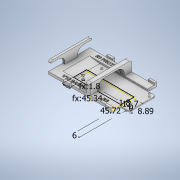
# Autodesk Inventor part: R1 Proto V10 Base
Saved by Autodesk Inventor 2021 (Build 250183000, 183)
## iProperties
Created: 2020-06-07
Part Number: R1 Proto V10 Base
Material: Generic
Document SubType Name: Modeling
Designer: andre
Density: 1 g/cm^3
Appearance: Default
Author: andre
## iProperties of the stored document _3DPrint.ipt
Created: 2020-06-07
Part Number: _3DPrint
Material: Generic
Document SubType Name: Modeling
Designer: andre
Density: 1 g/cm^3
Appearance: Default
Author: andre
Autodesk Inventor part; units mm, degrees
ref_plane "YZ Plane" through (0, 0, 0) normal (1, 0, 0) x (0, 1, 0)
ref_plane "XZ Plane" through (0, 0, 0) normal (0, 1, 0) x (-1, 0, 0)
ref_plane "XY Plane" through (0, 0, 0) normal (0, 0, 1) x (1, 0, 0)
sketch "Sketch1" plane through (0, 0, 0) normal (0, 1, 0) x (-1, 0, 0)
  line L0 (0, 0) -> (62, 0)
  line L1 (62, 0) -> (62, -19.7)
  line L2 (62, -19.7) -> (0, -19.7)
  line L3 (0, -19.7) -> (0, 0)
  dimension "d5" = 62
  dimension "d6" = 19.7
  constraints: 8 end point, 2 parallel, 1 horizontal, 1 perpendicular
  measures "d5" distance of L1.end L2.end
  measures "d6" distance of L0.end L1.end
extrude "Extrusion1" add sketch "Sketch1" along normal blind 2.4
sketch "Sketch3" plane through (-62, 0, 0) normal (0, 0, 1) x (1, 0, 0)
  line L0 (62, 2.4) -> (0, 2.4) projected
  line L1 (62, 0) -> (0, 0) projected
  line L2 (62, 2.4) -> (56, 2.4)
  line L3 (56, 2.4) -> (56, 0)
  line L4 (56, 0) -> (62, 0)
  line L5 (62, 0) -> (62, 2.4)
  line L6 (22, 2.4) -> (22, 0) construction
  line L7 (22, 2.4) -> (16, 2.4)
  line L8 (16, 2.4) -> (16, 0)
  line L9 (16, 0) -> (22, 0)
  line L10 (22, 0) -> (22, 2.4)
  point P0 (62, 0)
  point P1 (22, 0)
  dimension "d9" = 6
  dimension "d13" = 6
  dimension "d14" = 34
  dimension "d79" = 2.4
  constraints: 18 end point, 4 parallel, 4 point on line, 3 perpendicular, 2 horizontal
  measures "d9" distance of L4.end L3.end
  measures "d13" distance of L9.end L8.end
  measures "d14" distance between parallel lines of L3 L6
  measures "d79" distance between parallel lines of L1 L0
extrude "Extrusion2" add sketch "Sketch3" along normal blind 2 contours L5 L1 L3 L0 | L10 L1 L8 L0
ref_plane "Work Plane1" through (0, 0, -19.7) normal (0, 0, -1) x (-1, 0, 0)
sketch "Sketch4" plane through (0, 2.4, 0) normal (0, 1, 0) x (1, 0, 0)
  line L0 (-6, -2) -> (0, -2) projected
  line L1 (-6, -2) -> (0, -2)
  line L2 (0, -2) -> (0, 0)
  line L3 (0, 0) -> (-6, 0)
  line L4 (-6, 0) -> (-6, -2)
  line L5 (-46, -2) -> (-40, -2) projected
  line L6 (-40, 0) -> (-40, -2) projected
  line L7 (-46, -2) -> (-40, -2)
  line L8 (-40, -2) -> (-40, 0)
  line L9 (-40, 0) -> (-46, 0)
  line L10 (-46, 0) -> (-46, -2)
  constraints: 16 end point, 4 parallel, 2 horizontal, 2 perpendicular
extrude "Extrusion3" add sketch "Sketch4" along normal blind 1.6
sketch "Sketch5" plane through (0, 2.4, 0) normal (0, 1, 0) x (1, 0, 0)
  point P0 (0, 0)
sketch "Sketch6" plane through (0, 2.4, 0) normal (0, 1, 0) x (1, 0, 0)
  line L0 (0, 19.7) -> (-62, 19.7) projected
  line L1 (-40, 0) -> (-6, 0) projected
  line L2 (-22, 19.7) -> (-26, 19.7)
  line L3 (-26, 19.7) -> (-26, 0)
  line L4 (-26, 0) -> (-22, 0)
  line L5 (-22, 0) -> (-22, 19.7)
  line L6 (0, 19.7) -> (0, 0) projected
  point P0 (-22, 0)
  point P1 (-26, 19.7)
  dimension "d18" = 4
  dimension "d19" = 22
  constraints: 8 end point, 2 parallel, 2 point on line, 1 horizontal, 1 perpendicular
  measures "d18" distance of L4.end L3.end
  measures "d19" distance between parallel lines of L6 L5
extrude "Extrusion4" add sketch "Sketch6" along normal blind 9.6
sketch "Sketch7" plane through (-22, 2.4, 0) normal (1, 0, 0) x (0, 0, -1)
  point P0 (0, -2.4)
sketch "Sketch8" plane through (-22, 2.4, 0) normal (1, 0, 0) x (0, 0, -1)
  line L0 (19.7, 0) -> (19.7, 9.6) projected
  line L1 (19.7, 0) -> (7, 0)
  line L2 (7, 0) -> (7, 8.1)
  line L3 (7, 8.1) -> (19.7, 8.1)
  line L4 (19.7, 8.1) -> (19.7, 0)
  line L5 (0, 0) -> (0, 9.6) projected
  line L6 (19.7, 0) -> (0, 0) projected
  line L7 (0, 9.6) -> (19.7, 9.6) projected
  point P0 (0, -2.4)
  point P1 (19.7, 8.1)
  dimension "d22" = 19.7
  dimension "d23" = 9.6
  dimension "d24" = 12.7
  dimension "d25" = 8.1
  constraints: 8 end point, 2 parallel, 1 horizontal, 1 perpendicular
  measures "d22" distance between parallel lines of L0 L5
  measures "d23" distance between parallel lines of L6 L7
  measures "d24" distance between parallel lines of L0 L2
  measures "d25" distance between parallel lines of L1 L3
extrude "Extrusion5" cut sketch "Sketch8" against normal blind 37.6 contours L1 L2 L3 L0
ref_plane "Work Plane2" through (-43, 0, -19.7) normal (-1, 0, 0) x (0, 0, 1)
sketch "Sketch12" plane through (0, 2.4, 0) normal (0, 1, 0) x (1, 0, 0)
  line L0 (0, 19.7) -> (0, -2) projected
  line L1 (0, 19.7) -> (-45.34, 19.7)
  line L2 (-45.34, 19.7) -> (-45.34, 7)
  line L3 (-45.34, 7) -> (0, 7)
  line L4 (0, 7) -> (0, 19.7)
  point P0 (0, 0)
  point P1 (0, 7)
  dimension "d41" = 45.34
  dimension "d42" = 12.7
  constraints: 8 end point, 2 parallel, 1 horizontal, 1 perpendicular
  measures "d41" distance between parallel lines of L2 L0
  measures "d42" distance between parallel lines of L1 L3
extrude "Extrusion8" cut sketch "Sketch12" against normal blind 1.4
fillet "Fillet3" radius 2 1 edges at (-24, 12, 0) curvature continuous yes
fillet "Fillet4" radius 7 1 edges at (-24, 10.5, -7) curvature continuous yes
sketch "Sketch13" plane through (0, 1, 0) normal (0, 1, 0) x (1, 0, 0)
  circle A0 centre (6, 10.81) radius 0.9
  circle A1 centre (-39.72, 10.81) radius 0.9
  line L0 (-45.34, 19.7) -> (0, 19.7) projected
  line L1 (0, 19.7) -> (0, 7) projected
  point P0 (0, 0)
  dimension "d48" = 1.8
  dimension "d49" = 1.8
  dimension "d50" = 45.72
  dimension "d51" = 8.89
  dimension "d76" = 6
  dimension "d100" = 0
  constraints: 2 centre point
  measures "d48" diameter of A0
  measures "d49" diameter of A1
  measures "d50" distance of A1.centre A0.centre
  measures "d51" distance from line of L0 A0.centre
  measures "d76" distance from line of L1 A0.centre
  measures "d100" vertical distance of A0.centre A1.centre
extrude "Extrusion9" add sketch "Sketch13" along normal blind 3 contours A0
mirror "Mirror3" about plane through (0, 0, -19.7) normal (0, 0, -1) of "Extrusion4", "Extrusion5", "Fillet4", "Fillet3", "Extrusion1", "Extrusion3", "Extrusion2", "Extrusion9", "Extrusion8"
chamfer "Chamfer1" distance 10 distance2 1.4 1 edges at (-45.34, 2.4, -19.7) measured on face at (-45.84, 2.4, -19.7)
sketch "Sketch15" plane through (0, 2.4, 0) normal (0, 1, 0) x (1, 0, 0)
  line L0 (-57, 38.4) -> (-28, 38.4) construction
  line L1 (-28, 38.4) -> (-28, 33.2) construction
  line L2 (-28, 33.2) -> (-57, 33.2) construction
  line L3 (-57, 33.2) -> (-57, 38.4) construction
  line L4 (-59, 37.4) -> (-59, 2) projected
  line L5 (-26, 2) -> (-26, 37.4) projected
  line L6 (-22, 39.4) -> (-46, 39.4) projected
  line L7 (-55.34, 32.2) -> (0, 32.2) projected
  line L8 (-57, 6) -> (-28, 6) construction
  line L9 (-28, 6) -> (-28, 1) construction
  line L10 (-28, 1) -> (-57, 1) construction
  line L11 (-57, 1) -> (-57, 6) construction
  line L12 (0, 7) -> (-55.34, 7) projected
  line L13 (-40, 0) -> (-46, 0) projected
  line L14 (-15.9129, 6) -> (-6.0871, 6) construction
  line L15 (-6.0871, 6) -> (-6.0871, 1) construction
  line L16 (-6.0871, 1) -> (-15.9129, 1) construction
  line L17 (-15.9129, 1) -> (-15.9129, 6) construction
  line L18 (-22, 2) -> (-22, 37.4) projected
  line L19 (0, 7) -> (0, 0) projected
  spline S0 degree 2 poles (-50.5157, 2) (-50.3394, 2) (-50.1147, 2.1691) (-50.0495, 2.3527) knots 0 0 0 1 2 2 2
  line L20 (-50.0495, 2.3527) -> (-49.2307, 4.5556)
  spline S1 degree 2 poles (-49.2307, 4.5556) (-49.2017, 4.6377) (-49.2017, 4.7174) knots 0 0 0 1 1 1
  spline S2 degree 2 poles (-49.2017, 4.7174) (-49.2041, 4.8454) (-49.3732, 4.9976) (-49.5157, 5) knots 0 0 0 1 2 2 2
  spline S3 degree 2 poles (-49.5157, 5) (-49.6341, 5) (-49.779, 4.8865) (-49.8176, 4.7657) knots 0 0 0 1 2 2 2
  line L21 (-49.8176, 4.7657) -> (-50.4988, 2.6691)
  line L22 (-50.4988, 2.6691) -> (-50.5133, 2.6691)
  line L23 (-50.5133, 2.6691) -> (-51.1969, 4.7585)
  spline S4 degree 2 poles (-51.1969, 4.7585) (-51.2331, 4.8841) (-51.3853, 5) (-51.5085, 5) knots 0 0 0 1 2 2 2
  spline S5 degree 2 poles (-51.5085, 5) (-51.6558, 4.9976) (-51.8273, 4.8406) (-51.8297, 4.7101) knots 0 0 0 1 2 2 2
  spline S6 degree 2 poles (-51.8297, 4.7101) (-51.8297, 4.6232) (-51.8007, 4.5386) knots 0 0 0 1 1 1
  line L24 (-51.8007, 4.5386) -> (-50.9867, 2.3551)
  spline S7 degree 2 poles (-50.9867, 2.3551) (-50.9215, 2.1691) (-50.6944, 2) (-50.5157, 2) knots 0 0 0 1 2 2 2
  spline S8 degree 2 poles (-47.8708, 1.9952) (-47.7331, 1.9976) (-47.5713, 2.1618) (-47.5688, 2.3019) knots 0 0 0 1 2 2 2
  line L25 (-47.5688, 2.3019) -> (-47.5688, 4.6618)
  spline S9 degree 2 poles (-47.5688, 4.6618) (-47.5713, 4.8213) (-47.7524, 5.0024) (-47.9167, 5.0048) knots 0 0 0 1 2 2 2
  spline S10 degree 2 poles (-47.9167, 5.0048) (-48.0085, 5.0048) (-48.1751, 4.9589) (-48.279, 4.8889) knots 0 0 0 1 2 2 2
  line L26 (-48.279, 4.8889) -> (-48.8587, 4.4879)
  spline S11 degree 2 poles (-48.8587, 4.4879) (-48.9287, 4.4372) (-48.9915, 4.3285) (-48.9915, 4.2585) knots 0 0 0 1 2 2 2
  spline S12 degree 2 poles (-48.9915, 4.2585) (-48.9891, 4.1594) (-48.8708, 4.0411) (-48.7766, 4.0411) knots 0 0 0 1 2 2 2
  spline S13 degree 2 poles (-48.7766, 4.0411) (-48.7307, 4.0411) (-48.6558, 4.0652) (-48.6147, 4.0942) knots 0 0 0 1 2 2 2
  line L27 (-48.6147, 4.0942) -> (-48.1872, 4.3937)
  line L28 (-48.1872, 4.3937) -> (-48.1751, 4.3937)
  line L29 (-48.1751, 4.3937) -> (-48.1751, 2.3019)
  spline S14 degree 2 poles (-48.1751, 2.3019) (-48.1727, 2.1618) (-48.0085, 1.9976) (-47.8708, 1.9952) knots 0 0 0 1 2 2 2
  spline S15 degree 2 poles (-45.7597, 1.9734) (-45.3877, 1.9758) (-44.8563, 2.3478) (-44.5713, 3.0314) (-44.5688, 3.5072) knots 0 0 0 1 2 3 3 3
  spline S16 degree 2 poles (-44.5688, 3.5072) (-44.5713, 3.9807) (-44.8563, 4.6594) (-45.3901, 5.0242) (-45.7597, 5.0266) knots 0 0 0 1 2 3 3 3
  spline S17 degree 2 poles (-45.7597, 5.0266) (-46.1292, 5.0242) (-46.663, 4.657) (-46.9505, 3.9783) (-46.9505, 3.5048) knots 0 0 0 1 2 3 3 3
  spline S18 degree 2 poles (-46.9505, 3.5048) (-46.9505, 3.029) (-46.663, 2.3454) (-46.1316, 1.9758) (-45.7597, 1.9734) knots 0 0 0 1 2 3 3 3
  spline S19 degree 2 poles (-45.7597, 2.4638) (-46.0326, 2.4662) (-46.3273, 3) (-46.3297, 3.5048) knots 0 0 0 1 2 2 2
  spline S20 degree 2 poles (-46.3297, 3.5048) (-46.3273, 4.0048) (-46.0278, 4.5338) (-45.7597, 4.5362) knots 0 0 0 1 2 2 2
  spline S21 degree 2 poles (-45.7597, 4.5362) (-45.4891, 4.5338) (-45.192, 4.0048) (-45.1896, 3.5048) knots 0 0 0 1 2 2 2
  spline S22 degree 2 poles (-45.1896, 3.5048) (-45.192, 3) (-45.4867, 2.4662) (-45.7597, 2.4638) knots 0 0 0 1 2 2 2
  line L30 (-43.035, 2.0386) -> (-42.0471, 2.0386)
  spline S23 degree 2 poles (-42.0471, 2.0386) (-41.5737, 2.0435) (-41.0423, 2.4855) (-41.0374, 2.8744) knots 0 0 0 1 2 2 2
  spline S24 degree 2 poles (-41.0374, 2.8744) (-41.0423, 3.1691) (-41.4215, 3.5531) (-41.7258, 3.5821) knots 0 0 0 1 2 2 2
  line L31 (-41.7258, 3.5821) -> (-41.7258, 3.5966)
  spline S25 degree 2 poles (-41.7258, 3.5966) (-41.4867, 3.6377) (-41.1824, 3.9855) (-41.1775, 4.2319) knots 0 0 0 1 2 2 2
  spline S26 degree 2 poles (-41.1775, 4.2319) (-41.18, 4.57) (-41.6534, 4.9565) (-42.0688, 4.9589) knots 0 0 0 1 2 2 2
  line L32 (-42.0688, 4.9589) -> (-43.035, 4.9589)
  spline S27 degree 2 poles (-43.035, 4.9589) (-43.18, 4.9589) (-43.3394, 4.7923) (-43.3394, 4.6425) knots 0 0 0 1 2 2 2
  line L33 (-43.3394, 4.6425) -> (-43.3394, 2.3575)
  spline S28 degree 2 poles (-43.3394, 2.3575) (-43.3394, 2.2053) (-43.18, 2.0386) (-43.035, 2.0386) knots 0 0 0 1 2 2 2
  line L34 (-42.7283, 2.4952) -> (-42.7283, 3.343)
  line L35 (-42.7283, 3.343) -> (-42.2162, 3.343)
  spline S29 degree 2 poles (-42.2162, 3.343) (-41.9457, 3.3406) (-41.6606, 3.128) (-41.6606, 2.9227) knots 0 0 0 1 2 2 2
  spline S30 degree 2 poles (-41.6606, 2.9227) (-41.6606, 2.7126) (-41.9384, 2.4952) (-42.2041, 2.4952) knots 0 0 0 1 2 2 2
  line L36 (-42.2041, 2.4952) -> (-42.7283, 2.4952)
  line L37 (-42.7283, 3.744) -> (-42.7283, 4.5048)
  line L38 (-42.7283, 4.5048) -> (-42.2283, 4.5048)
  spline S31 degree 2 poles (-42.2283, 4.5048) (-42.0109, 4.5024) (-41.779, 4.3116) (-41.779, 4.1353) knots 0 0 0 1 2 2 2
  spline S32 degree 2 poles (-41.779, 4.1353) (-41.779, 3.9493) (-42.0447, 3.7464) (-42.2911, 3.744) knots 0 0 0 1 2 2 2
  line L39 (-42.2911, 3.744) -> (-42.7283, 3.744)
  spline S33 degree 2 poles (-40.494, 2) (-40.3732, 2) (-40.2258, 2.1304) (-40.1848, 2.2754) knots 0 0 0 1 2 2 2
  line L40 (-40.1848, 2.2754) -> (-40.0302, 2.7319)
  line L41 (-40.0302, 2.7319) -> (-38.9771, 2.7319)
  line L42 (-38.9771, 2.7319) -> (-38.8225, 2.2705)
  spline S34 degree 2 poles (-38.8225, 2.2705) (-38.7814, 2.128) (-38.6316, 2) (-38.5036, 2) knots 0 0 0 1 2 2 2
  spline S35 degree 2 poles (-38.5036, 2) (-38.3684, 2.0024) (-38.2017, 2.1594) (-38.1993, 2.2874) knots 0 0 0 1 2 2 2
  spline S36 degree 2 poles (-38.1993, 2.2874) (-38.1993, 2.3333) (-38.2162, 2.4227) (-38.2379, 2.4831) knots 0 0 0 1 2 2 2
  line L43 (-38.2379, 2.4831) -> (-39.0399, 4.6546)
  spline S37 degree 2 poles (-39.0399, 4.6546) (-39.1027, 4.8333) (-39.3273, 5) (-39.506, 5) knots 0 0 0 1 2 2 2
  spline S38 degree 2 poles (-39.506, 5) (-39.6775, 5) (-39.9022, 4.8309) (-39.965, 4.6546) knots 0 0 0 1 2 2 2
  line L44 (-39.965, 4.6546) -> (-40.7621, 2.4831)
  spline S39 degree 2 poles (-40.7621, 2.4831) (-40.7838, 2.4251) (-40.8031, 2.3261) (-40.8031, 2.2874) knots 0 0 0 1 2 2 2
  spline S40 degree 2 poles (-40.8031, 2.2874) (-40.8031, 2.1546) (-40.6389, 2.0024) (-40.494, 2) knots 0 0 0 1 2 2 2
  line L45 (-39.8973, 3.2053) -> (-39.5181, 4.401)
  line L46 (-39.5181, 4.401) -> (-39.5036, 4.401)
  line L47 (-39.5036, 4.401) -> (-39.1171, 3.2053)
  line L48 (-39.1171, 3.2053) -> (-39.8973, 3.2053)
  spline S41 degree 2 poles (-36.7597, 1.9903) (-36.2089, 1.9952) (-35.5882, 2.4879) (-35.5833, 2.9203) knots 0 0 0 1 2 2 2
  spline S42 degree 2 poles (-35.5833, 2.9203) (-35.5809, 3.2512) (-36.0085, 3.6473) (-36.4698, 3.7367) knots 0 0 0 1 2 2 2
  line L49 (-36.4698, 3.7367) -> (-36.779, 3.7995)
  spline S43 degree 2 poles (-36.779, 3.7995) (-37.035, 3.8502) (-37.2669, 4.0266) (-37.2645, 4.1594) knots 0 0 0 1 2 2 2
  spline S44 degree 2 poles (-37.2645, 4.1594) (-37.2597, 4.3237) (-36.9915, 4.5145) (-36.7621, 4.5169) knots 0 0 0 1 2 2 2
  spline S45 degree 2 poles (-36.7621, 4.5169) (-36.5737, 4.5169) (-36.2983, 4.3696) (-36.2258, 4.2053) knots 0 0 0 1 2 2 2
  spline S46 degree 2 poles (-36.2258, 4.2053) (-36.1751, 4.1111) (-36.035, 4.0242) (-35.9336, 4.0242) knots 0 0 0 1 2 2 2
  spline S47 degree 2 poles (-35.9336, 4.0242) (-35.8152, 4.0266) (-35.6751, 4.1594) (-35.6727, 4.2681) knots 0 0 0 1 2 2 2
  spline S48 degree 2 poles (-35.6727, 4.2681) (-35.6727, 4.3092) (-35.6848, 4.3744) (-35.6944, 4.4058) knots 0 0 0 1 2 2 2
  spline S49 degree 2 poles (-35.6944, 4.4058) (-35.7959, 4.6932) (-36.3563, 5.0072) (-36.7621, 5.0097) knots 0 0 0 1 2 2 2
  spline S50 degree 2 poles (-36.7621, 5.0097) (-37.0882, 5.0072) (-37.5906, 4.7874) (-37.8732, 4.3913) (-37.878, 4.1208) knots 0 0 0 1 2 3 3 3
  spline S51 degree 2 poles (-37.878, 4.1208) (-37.878, 3.7947) (-37.4457, 3.3792) (-37.0085, 3.2923) knots 0 0 0 1 2 2 2
  line L50 (-37.0085, 3.2923) -> (-36.6993, 3.2319)
  spline S52 degree 2 poles (-36.6993, 3.2319) (-36.4263, 3.1763) (-36.192, 2.9976) (-36.1944, 2.8551) knots 0 0 0 1 2 2 2
  spline S53 degree 2 poles (-36.1944, 2.8551) (-36.1993, 2.6908) (-36.4964, 2.4855) (-36.7452, 2.4831) knots 0 0 0 1 2 2 2
  spline S54 degree 2 poles (-36.7452, 2.4831) (-36.9577, 2.4807) (-37.2742, 2.6401) (-37.349, 2.8068) knots 0 0 0 1 2 2 2
  spline S55 degree 2 poles (-37.349, 2.8068) (-37.4022, 2.901) (-37.5374, 2.9855) (-37.6292, 2.9831) knots 0 0 0 1 2 2 2
  spline S56 degree 2 poles (-37.6292, 2.9831) (-37.75, 2.9831) (-37.8973, 2.8382) (-37.8998, 2.715) knots 0 0 0 1 2 2 2
  spline S57 degree 2 poles (-37.8998, 2.715) (-37.8998, 2.6739) (-37.8829, 2.5894) (-37.8659, 2.5507) knots 0 0 0 1 2 2 2
  spline S58 degree 2 poles (-37.8659, 2.5507) (-37.7766, 2.3068) (-37.2138, 1.9952) (-36.7597, 1.9903) knots 0 0 0 1 2 2 2
  line L51 (-34.907, 2.0386) -> (-33.5181, 2.0386)
  spline S59 degree 2 poles (-33.5181, 2.0386) (-33.3901, 2.0386) (-33.2428, 2.1715) (-33.2403, 2.2923) knots 0 0 0 1 2 2 2
  spline S60 degree 2 poles (-33.2403, 2.2923) (-33.2428, 2.4106) (-33.3925, 2.5435) (-33.5181, 2.5435) knots 0 0 0 1 2 2 2
  line L52 (-33.5181, 2.5435) -> (-34.6002, 2.5435)
  line L53 (-34.6002, 2.5435) -> (-34.6002, 3.2826)
  line L54 (-34.6002, 3.2826) -> (-33.5713, 3.2826)
  spline S61 degree 2 poles (-33.5713, 3.2826) (-33.4529, 3.2826) (-33.3176, 3.4058) (-33.3152, 3.5169) knots 0 0 0 1 2 2 2
  spline S62 degree 2 poles (-33.3152, 3.5169) (-33.3176, 3.6256) (-33.4553, 3.7512) (-33.5713, 3.7512) knots 0 0 0 1 2 2 2
  line L55 (-33.5713, 3.7512) -> (-34.6002, 3.7512)
  line L56 (-34.6002, 3.7512) -> (-34.6002, 4.4541)
  line L57 (-34.6002, 4.4541) -> (-33.5181, 4.4541)
  spline S63 degree 2 poles (-33.5181, 4.4541) (-33.3925, 4.4541) (-33.2428, 4.587) (-33.2403, 4.7053) knots 0 0 0 1 2 2 2
  spline S64 degree 2 poles (-33.2403, 4.7053) (-33.2428, 4.8261) (-33.3901, 4.9589) (-33.5181, 4.9589) knots 0 0 0 1 2 2 2
  line L58 (-33.5181, 4.9589) -> (-34.907, 4.9589)
  spline S65 degree 2 poles (-34.907, 4.9589) (-35.0519, 4.9589) (-35.2114, 4.7923) (-35.2114, 4.6425) knots 0 0 0 1 2 2 2
  line L59 (-35.2114, 4.6425) -> (-35.2114, 2.3575)
  spline S66 degree 2 poles (-35.2114, 2.3575) (-35.2114, 2.2053) (-35.0519, 2.0386) (-34.907, 2.0386) knots 0 0 0 1 2 2 2
  spline S67 degree 2 poles (-51.6534, 34.2952) (-51.5085, 34.2976) (-51.349, 34.4618) (-51.3466, 34.614) knots 0 0 0 1 2 2 2
  line L60 (-51.3466, 34.614) -> (-51.3466, 35.4063)
  line L61 (-51.3466, 35.4063) -> (-50.8273, 35.4063)
  line L62 (-50.8273, 35.4063) -> (-50.3418, 34.5271)
  spline S68 degree 2 poles (-50.3418, 34.5271) (-50.2717, 34.3966) (-50.1365, 34.2928) (-50.0302, 34.2952) knots 0 0 0 1 2 2 2
  spline S69 degree 2 poles (-50.0302, 34.2952) (-49.8949, 34.2976) (-49.7258, 34.4522) (-49.721, 34.5754) knots 0 0 0 1 2 2 2
  spline S70 degree 2 poles (-49.721, 34.5754) (-49.721, 34.6261) (-49.75, 34.7227) (-49.7862, 34.7855) knots 0 0 0 1 2 2 2
  line L63 (-49.7862, 34.7855) -> (-50.2089, 35.515)
  spline S71 degree 2 poles (-50.2089, 35.515) (-49.965, 35.6213) (-49.7065, 36.0512) (-49.7065, 36.329) knots 0 0 0 1 2 2 2
  spline S72 degree 2 poles (-49.7065, 36.329) (-49.7089, 36.7662) (-50.2548, 37.2541) (-50.7621, 37.2589) knots 0 0 0 1 2 2 2
  line L64 (-50.7621, 37.2589) -> (-51.6534, 37.2589)
  spline S73 degree 2 poles (-51.6534, 37.2589) (-51.7983, 37.2589) (-51.9577, 37.0923) (-51.9577, 36.9425) knots 0 0 0 1 2 2 2
  line L65 (-51.9577, 36.9425) -> (-51.9577, 34.614)
  spline S74 degree 2 poles (-51.9577, 34.614) (-51.9577, 34.4618) (-51.7983, 34.2976) (-51.6534, 34.2952) knots 0 0 0 1 2 2 2
  line L66 (-51.3466, 35.8507) -> (-51.3466, 36.7807)
  line L67 (-51.3466, 36.7807) -> (-50.8273, 36.7807)
  spline S75 degree 2 poles (-50.8273, 36.7807) (-50.5978, 36.7783) (-50.337, 36.5319) (-50.3345, 36.3169) knots 0 0 0 1 2 2 2
  spline S76 degree 2 poles (-50.3345, 36.3169) (-50.3345, 36.0971) (-50.5882, 35.8531) (-50.8225, 35.8507) knots 0 0 0 1 2 2 2
  line L68 (-50.8225, 35.8507) -> (-51.3466, 35.8507)
  spline S77 degree 2 poles (-48.3104, 34.2952) (-48.1727, 34.2976) (-48.0109, 34.4618) (-48.0085, 34.6019) knots 0 0 0 1 2 2 2
  line L69 (-48.0085, 34.6019) -> (-48.0085, 36.9618)
  spline S78 degree 2 poles (-48.0085, 36.9618) (-48.0109, 37.1213) (-48.192, 37.3024) (-48.3563, 37.3048) knots 0 0 0 1 2 2 2
  spline S79 degree 2 poles (-48.3563, 37.3048) (-48.4481, 37.3048) (-48.6147, 37.2589) (-48.7186, 37.1889) knots 0 0 0 1 2 2 2
  line L70 (-48.7186, 37.1889) -> (-49.2983, 36.7879)
  spline S80 degree 2 poles (-49.2983, 36.7879) (-49.3684, 36.7372) (-49.4312, 36.6285) (-49.4312, 36.5585) knots 0 0 0 1 2 2 2
  spline S81 degree 2 poles (-49.4312, 36.5585) (-49.4287, 36.4594) (-49.3104, 36.3411) (-49.2162, 36.3411) knots 0 0 0 1 2 2 2
  spline S82 degree 2 poles (-49.2162, 36.3411) (-49.1703, 36.3411) (-49.0954, 36.3652) (-49.0543, 36.3942) knots 0 0 0 1 2 2 2
  line L71 (-49.0543, 36.3942) -> (-48.6268, 36.6937)
  line L72 (-48.6268, 36.6937) -> (-48.6147, 36.6937)
  line L73 (-48.6147, 36.6937) -> (-48.6147, 34.6019)
  spline S83 degree 2 poles (-48.6147, 34.6019) (-48.6123, 34.4618) (-48.4481, 34.2976) (-48.3104, 34.2952) knots 0 0 0 1 2 2 2
  spline S84 degree 2 poles (-46.192, 34.3) (-46.0471, 34.3024) (-45.8877, 34.4667) (-45.8853, 34.6188) knots 0 0 0 1 2 2 2
  line L74 (-45.8853, 34.6188) -> (-45.8853, 35.2589)
  line L75 (-45.8853, 35.2589) -> (-45.3394, 35.2589)
  spline S85 degree 2 poles (-45.3394, 35.2589) (-45.0302, 35.2614) (-44.5616, 35.5101) (-44.2983, 35.957) (-44.2983, 36.2589) knots 0 0 0 1 2 3 3 3
  spline S86 degree 2 poles (-44.2983, 36.2589) (-44.2983, 36.5609) (-44.5543, 37.0101) (-45.0085, 37.2565) (-45.3104, 37.2589) knots 0 0 0 1 2 3 3 3
  line L76 (-45.3104, 37.2589) -> (-46.192, 37.2589)
  spline S87 degree 2 poles (-46.192, 37.2589) (-46.337, 37.2589) (-46.4964, 37.0923) (-46.4964, 36.9425) knots 0 0 0 1 2 2 2
  line L77 (-46.4964, 36.9425) -> (-46.4964, 34.6188)
  spline S88 degree 2 poles (-46.4964, 34.6188) (-46.4964, 34.4667) (-46.337, 34.3024) (-46.192, 34.3) knots 0 0 0 1 2 2 2
  line L78 (-45.8853, 35.7372) -> (-45.8853, 36.7758)
  line L79 (-45.8853, 36.7758) -> (-45.4722, 36.7758)
  spline S89 degree 2 poles (-45.4722, 36.7758) (-45.2065, 36.7734) (-44.9215, 36.5077) (-44.9191, 36.2565) knots 0 0 0 1 2 2 2
  spline S90 degree 2 poles (-44.9191, 36.2565) (-44.9215, 36.0053) (-45.2089, 35.7396) (-45.4722, 35.7372) knots 0 0 0 1 2 2 2
  line L80 (-45.4722, 35.7372) -> (-45.8853, 35.7372)
  spline S91 degree 2 poles (-43.6316, 34.2952) (-43.4867, 34.2976) (-43.3273, 34.4618) (-43.3249, 34.614) knots 0 0 0 1 2 2 2
  line L81 (-43.3249, 34.614) -> (-43.3249, 35.4063)
  line L82 (-43.3249, 35.4063) -> (-42.8056, 35.4063)
  line L83 (-42.8056, 35.4063) -> (-42.32, 34.5271)
  spline S92 degree 2 poles (-42.32, 34.5271) (-42.25, 34.3966) (-42.1147, 34.2928) (-42.0085, 34.2952) knots 0 0 0 1 2 2 2
  spline S93 degree 2 poles (-42.0085, 34.2952) (-41.8732, 34.2976) (-41.7041, 34.4522) (-41.6993, 34.5754) knots 0 0 0 1 2 2 2
  spline S94 degree 2 poles (-41.6993, 34.5754) (-41.6993, 34.6261) (-41.7283, 34.7227) (-41.7645, 34.7855) knots 0 0 0 1 2 2 2
  line L84 (-41.7645, 34.7855) -> (-42.1872, 35.515)
  spline S95 degree 2 poles (-42.1872, 35.515) (-41.9432, 35.6213) (-41.6848, 36.0512) (-41.6848, 36.329) knots 0 0 0 1 2 2 2
  spline S96 degree 2 poles (-41.6848, 36.329) (-41.6872, 36.7662) (-42.2331, 37.2541) (-42.7403, 37.2589) knots 0 0 0 1 2 2 2
  line L85 (-42.7403, 37.2589) -> (-43.6316, 37.2589)
  spline S97 degree 2 poles (-43.6316, 37.2589) (-43.7766, 37.2589) (-43.936, 37.0923) (-43.936, 36.9425) knots 0 0 0 1 2 2 2
  line L86 (-43.936, 36.9425) -> (-43.936, 34.614)
  spline S98 degree 2 poles (-43.936, 34.614) (-43.936, 34.4618) (-43.7766, 34.2976) (-43.6316, 34.2952) knots 0 0 0 1 2 2 2
  line L87 (-43.3249, 35.8507) -> (-43.3249, 36.7807)
  line L88 (-43.3249, 36.7807) -> (-42.8056, 36.7807)
  spline S99 degree 2 poles (-42.8056, 36.7807) (-42.5761, 36.7783) (-42.3152, 36.5319) (-42.3128, 36.3169) knots 0 0 0 1 2 2 2
  spline S100 degree 2 poles (-42.3128, 36.3169) (-42.3128, 36.0971) (-42.5664, 35.8531) (-42.8007, 35.8507) knots 0 0 0 1 2 2 2
  line L89 (-42.8007, 35.8507) -> (-43.3249, 35.8507)
  spline S101 degree 2 poles (-39.9674, 34.2903) (-39.5326, 34.2928) (-38.9022, 34.6575) (-38.5616, 35.3314) (-38.5592, 35.7976) knots 0 0 0 1 2 3 3 3
  spline S102 degree 2 poles (-38.5592, 35.7976) (-38.5616, 36.2662) (-38.9022, 36.9425) (-39.5326, 37.3072) (-39.9674, 37.3097) knots 0 0 0 1 2 3 3 3
  spline S103 degree 2 poles (-39.9674, 37.3097) (-40.4022, 37.3072) (-41.0326, 36.9425) (-41.3732, 36.2662) (-41.3756, 35.7976) knots 0 0 0 1 2 3 3 3
  spline S104 degree 2 poles (-41.3756, 35.7976) (-41.3732, 35.3314) (-41.0326, 34.6575) (-40.4022, 34.2928) (-39.9674, 34.2903) knots 0 0 0 1 2 3 3 3
  spline S105 degree 2 poles (-39.9674, 34.8) (-40.3321, 34.8048) (-40.7476, 35.3338) (-40.7524, 35.7976) knots 0 0 0 1 2 2 2
  spline S106 degree 2 poles (-40.7524, 35.7976) (-40.7476, 36.2638) (-40.3297, 36.7952) (-39.9674, 36.8) knots 0 0 0 1 2 2 2
  spline S107 degree 2 poles (-39.9674, 36.8) (-39.6051, 36.7952) (-39.1872, 36.2638) (-39.1848, 35.7976) knots 0 0 0 1 2 2 2
  spline S108 degree 2 poles (-39.1848, 35.7976) (-39.1872, 35.3338) (-39.6051, 34.8048) (-39.9674, 34.8) knots 0 0 0 1 2 2 2
  spline S109 degree 2 poles (-37.163, 34.3) (-37.0181, 34.3024) (-36.8587, 34.4667) (-36.8563, 34.6188) knots 0 0 0 1 2 2 2
  line L90 (-36.8563, 34.6188) -> (-36.8563, 36.7541)
  line L91 (-36.8563, 36.7541) -> (-36.2524, 36.7541)
  spline S110 degree 2 poles (-36.2524, 36.7541) (-36.1268, 36.7541) (-35.9795, 36.887) (-35.9771, 37.0053) knots 0 0 0 1 2 2 2
  spline S111 degree 2 poles (-35.9771, 37.0053) (-35.9771, 37.1261) (-36.1268, 37.2589) (-36.2524, 37.2589) knots 0 0 0 1 2 2 2
  line L92 (-36.2524, 37.2589) -> (-38.0713, 37.2589)
  spline S112 degree 2 poles (-38.0713, 37.2589) (-38.1993, 37.2589) (-38.3466, 37.1261) (-38.349, 37.0053) knots 0 0 0 1 2 2 2
  spline S113 degree 2 poles (-38.349, 37.0053) (-38.3466, 36.887) (-38.1969, 36.7541) (-38.0713, 36.7541) knots 0 0 0 1 2 2 2
  line L93 (-38.0713, 36.7541) -> (-37.4674, 36.7541)
  line L94 (-37.4674, 36.7541) -> (-37.4674, 34.6188)
  spline S114 degree 2 poles (-37.4674, 34.6188) (-37.4674, 34.4667) (-37.308, 34.3024) (-37.163, 34.3) knots 0 0 0 1 2 2 2
  spline S115 degree 2 poles (-34.3563, 34.2903) (-33.9215, 34.2928) (-33.2911, 34.6575) (-32.9505, 35.3314) (-32.9481, 35.7976) knots 0 0 0 1 2 3 3 3
  spline S116 degree 2 poles (-32.9481, 35.7976) (-32.9505, 36.2662) (-33.2911, 36.9425) (-33.9215, 37.3072) (-34.3563, 37.3097) knots 0 0 0 1 2 3 3 3
  spline S117 degree 2 poles (-34.3563, 37.3097) (-34.7911, 37.3072) (-35.4215, 36.9425) (-35.7621, 36.2662) (-35.7645, 35.7976) knots 0 0 0 1 2 3 3 3
  spline S118 degree 2 poles (-35.7645, 35.7976) (-35.7621, 35.3314) (-35.4215, 34.6575) (-34.7911, 34.2928) (-34.3563, 34.2903) knots 0 0 0 1 2 3 3 3
  spline S119 degree 2 poles (-34.3563, 34.8) (-34.721, 34.8048) (-35.1365, 35.3338) (-35.1413, 35.7976) knots 0 0 0 1 2 2 2
  spline S120 degree 2 poles (-35.1413, 35.7976) (-35.1365, 36.2638) (-34.7186, 36.7952) (-34.3563, 36.8) knots 0 0 0 1 2 2 2
  spline S121 degree 2 poles (-34.3563, 36.8) (-33.994, 36.7952) (-33.5761, 36.2638) (-33.5737, 35.7976) knots 0 0 0 1 2 2 2
  spline S122 degree 2 poles (-33.5737, 35.7976) (-33.5761, 35.3338) (-33.994, 34.8048) (-34.3563, 34.8) knots 0 0 0 1 2 2 2
  line L95 (-13.0833, 2.0386) -> (-12.0954, 2.0386)
  spline S123 degree 2 poles (-12.0954, 2.0386) (-11.622, 2.0435) (-11.0906, 2.4855) (-11.0857, 2.8744) knots 0 0 0 1 2 2 2
  spline S124 degree 2 poles (-11.0857, 2.8744) (-11.0906, 3.1691) (-11.4698, 3.5531) (-11.7742, 3.5821) knots 0 0 0 1 2 2 2
  line L96 (-11.7742, 3.5821) -> (-11.7742, 3.5966)
  spline S125 degree 2 poles (-11.7742, 3.5966) (-11.535, 3.6377) (-11.2307, 3.9855) (-11.2258, 4.2319) knots 0 0 0 1 2 2 2
  spline S126 degree 2 poles (-11.2258, 4.2319) (-11.2283, 4.57) (-11.7017, 4.9565) (-12.1171, 4.9589) knots 0 0 0 1 2 2 2
  line L97 (-12.1171, 4.9589) -> (-13.0833, 4.9589)
  spline S127 degree 2 poles (-13.0833, 4.9589) (-13.2283, 4.9589) (-13.3877, 4.7923) (-13.3877, 4.6425) knots 0 0 0 1 2 2 2
  line L98 (-13.3877, 4.6425) -> (-13.3877, 2.3575)
  spline S128 degree 2 poles (-13.3877, 2.3575) (-13.3877, 2.2053) (-13.2283, 2.0386) (-13.0833, 2.0386) knots 0 0 0 1 2 2 2
  line L99 (-12.7766, 2.4952) -> (-12.7766, 3.343)
  line L100 (-12.7766, 3.343) -> (-12.2645, 3.343)
  spline S129 degree 2 poles (-12.2645, 3.343) (-11.994, 3.3406) (-11.7089, 3.128) (-11.7089, 2.9227) knots 0 0 0 1 2 2 2
  spline S130 degree 2 poles (-11.7089, 2.9227) (-11.7089, 2.7126) (-11.9867, 2.4952) (-12.2524, 2.4952) knots 0 0 0 1 2 2 2
  line L101 (-12.2524, 2.4952) -> (-12.7766, 2.4952)
  line L102 (-12.7766, 3.744) -> (-12.7766, 4.5048)
  line L103 (-12.7766, 4.5048) -> (-12.2766, 4.5048)
  spline S131 degree 2 poles (-12.2766, 4.5048) (-12.0592, 4.5024) (-11.8273, 4.3116) (-11.8273, 4.1353) knots 0 0 0 1 2 2 2
  spline S132 degree 2 poles (-11.8273, 4.1353) (-11.8273, 3.9493) (-12.093, 3.7464) (-12.3394, 3.744) knots 0 0 0 1 2 2 2
  line L104 (-12.3394, 3.744) -> (-12.7766, 3.744)
  spline S133 degree 2 poles (-9.6872, 1.9734) (-9.3466, 1.9758) (-8.837, 2.1932) (-8.5519, 2.5894) (-8.5495, 2.8575) knots 0 0 0 1 2 3 3 3
  spline S134 degree 2 poles (-8.5495, 2.8575) (-8.5543, 3.1594) (-8.936, 3.5217) (-9.2669, 3.5556) knots 0 0 0 1 2 2 2
  line L105 (-9.2669, 3.5556) -> (-9.2669, 3.5676)
  spline S135 degree 2 poles (-9.2669, 3.5676) (-9.0036, 3.6208) (-8.663, 3.971) (-8.6582, 4.2512) knots 0 0 0 1 2 2 2
  spline S136 degree 2 poles (-8.6582, 4.2512) (-8.6606, 4.4855) (-8.9167, 4.8333) (-9.3804, 5.0217) (-9.692, 5.0242) knots 0 0 0 1 2 3 3 3
  spline S137 degree 2 poles (-9.692, 5.0242) (-10.0809, 5.0193) (-10.5713, 4.7198) (-10.6703, 4.5) knots 0 0 0 1 2 2 2
  spline S138 degree 2 poles (-10.6703, 4.5) (-10.692, 4.4493) (-10.7138, 4.3551) (-10.7138, 4.3043) knots 0 0 0 1 2 2 2
  spline S139 degree 2 poles (-10.7138, 4.3043) (-10.7138, 4.1908) (-10.5857, 4.058) (-10.4577, 4.0556) knots 0 0 0 1 2 2 2
  spline S140 degree 2 poles (-10.4577, 4.0556) (-10.3563, 4.0556) (-10.2307, 4.1425) (-10.1824, 4.244) knots 0 0 0 1 2 2 2
  spline S141 degree 2 poles (-10.1824, 4.244) (-10.1123, 4.3986) (-9.8732, 4.5556) (-9.6896, 4.5556) knots 0 0 0 1 2 2 2
  spline S142 degree 2 poles (-9.6896, 4.5556) (-9.4674, 4.5531) (-9.2379, 4.343) (-9.2379, 4.1643) knots 0 0 0 1 2 2 2
  spline S143 degree 2 poles (-9.2379, 4.1643) (-9.2403, 3.9831) (-9.5085, 3.7609) (-9.7403, 3.7585) knots 0 0 0 1 2 2 2
  line L106 (-9.7403, 3.7585) -> (-9.8611, 3.7585)
  spline S144 degree 2 poles (-9.8611, 3.7585) (-9.9722, 3.7585) (-10.093, 3.6401) (-10.093, 3.5435) knots 0 0 0 1 2 2 2
  spline S145 degree 2 poles (-10.093, 3.5435) (-10.093, 3.442) (-9.9722, 3.3261) (-9.8611, 3.3237) knots 0 0 0 1 2 2 2
  line L107 (-9.8611, 3.3237) -> (-9.7331, 3.3237)
  spline S146 degree 2 poles (-9.7331, 3.3237) (-9.465, 3.3237) (-9.1727, 3.0966) (-9.1727, 2.8816) knots 0 0 0 1 2 2 2
  spline S147 degree 2 poles (-9.1727, 2.8816) (-9.1751, 2.6981) (-9.4505, 2.4686) (-9.6775, 2.4662) knots 0 0 0 1 2 2 2
  spline S148 degree 2 poles (-9.6775, 2.4662) (-9.9022, 2.4662) (-10.1679, 2.6377) (-10.2428, 2.7923) knots 0 0 0 1 2 2 2
  spline S149 degree 2 poles (-10.2428, 2.7923) (-10.2862, 2.8744) (-10.4118, 2.9517) (-10.5012, 2.9517) knots 0 0 0 1 2 2 2
  spline S150 degree 2 poles (-10.5012, 2.9517) (-10.6292, 2.9493) (-10.7693, 2.814) (-10.7717, 2.6957) knots 0 0 0 1 2 2 2
  spline S151 degree 2 poles (-10.7717, 2.6957) (-10.7717, 2.6498) (-10.7476, 2.5531) (-10.7234, 2.5024) knots 0 0 0 1 2 2 2
  spline S152 degree 2 poles (-10.7234, 2.5024) (-10.6558, 2.3575) (-10.3804, 2.1184) (-9.9674, 1.9758) (-9.6872, 1.9734) knots 0 0 0 1 2 3 3 3
  point P0 (-59, 39.4)
  point P1 (-55.34, 32.4)
  point P2 (0, 32.4)
  point P3 (-59, 0)
  dimension "d59" = 2
  dimension "d60" = 2
  dimension "d61" = 1
  dimension "d62" = 1
  dimension "d63" = 1
  dimension "d64" = 1
  dimension "d65" = 2
  dimension "d66" = 2
  dimension "d69" = 0
  dimension "d70" = 0
  dimension "d71" = 6.0871
  dimension "d72" = 6.0871
  constraints: 6 other
  measures "d59" distance between parallel lines of L4 L3
  measures "d60" distance between parallel lines of L5 L1
  measures "d61" distance between parallel lines of L6 L0
  measures "d62" distance between parallel lines of L7 L2
  measures "d63" distance between parallel lines of L12 L8
  measures "d64" distance between parallel lines of L13 L10
  measures "d65" distance between parallel lines of L4 L11
  measures "d66" distance between parallel lines of L5 L9
  measures "d69" distance between parallel lines of L14 L8
  measures "d70" distance between parallel lines of L16 L10
  measures "d71" distance between parallel lines of L18 L17
  measures "d72" distance between parallel lines of L19 L15
extrude "Extrusion11" cut sketch "Sketch15" against normal blind 1 contours S7 L24 S6 S5 S4 L23 L22 L21 S3 S2 S1 L20 S0 | S14 L29 L28 L27 S13 S12 S11 L26 S10 S9 L25 S8 | S18 S17 S16 S15 | S28 L33 S27 L32 S26 S25 L31 S24 S23 L30 | S40 S39 L44 S38 S37 L43 S36 S35 S34 L42 L41 L40 S33 | S58 S57 S56 S55 S54 S53 S52 L50 S51 S50 S49 S48 S47 S46 S45 S44 S43 L49 S42 S41 | S66 L59 S65 L58 S64 S63 L57 L56 L55 S62 S61 L54 L53 L52 S60 S59 L51 | S74 L65 S73 L64 S72 S71 L63 S70 S69 S68 L62 L61 L60 S67 | S83 L73 L72 L71 S82 S81 S80 L70 S79 S78 L69 S77 | S88 L77 S87 L76 S86 S85 L75 L74 S84 | S98 L86 S97 L85 S96 S95 L84 S94 S93 S92 L83 L82 L81 S91 | S104 S103 S102 S101 | S114 L94 L93 S113 S112 L92 S111 S110 L91 L90 S109 | S118 S117 S116 S115 | S128 L98 S127 L97 S126 S125 L96 S124 S123 L95 | S152 S151 S150 S149 S148 S147 S146 L107 S145 S144 L106 S143 S142 S141 S140 S139 S138 S137 S136 S135 L105 S134 S133
sketch "Sketch16" plane through (0, 0, 2) normal (1, 0, 0) x (0, 0, -1)
  line L0 (34.4, 1) -> (9, 1) projected
  line L1 (2, 0) -> (41.4, 0) projected
  line L2 (9, 1) -> (34.4, 1)
  line L3 (34.4, 1) -> (34.4, 0)
  line L4 (34.4, 0) -> (9, 0)
  line L5 (9, 0) -> (9, 1)
  point P0 (9, 0)
  dimension "d73" = 25.4
  constraints: 8 end point, 2 parallel, 1 horizontal, 1 perpendicular, 1 point on line
  measures "d73" distance of L3.end L4.end
extrude "Extrusion12" add sketch "Sketch16" along normal blind 8
extrude "Extrusion13" add sketch "Sketch13" along normal blind 1 contours A1
mirror "Mirror4" about plane through (0, 0, -19.7) normal (0, 0, -1) of "Extrusion13"
fillet "Fillet5" radius 2 2 edges at (8, 0.5, -7) (8, 0.5, -32.4) curvature continuous yes
sketch "Sketch18" plane through (0, 2.4, 0) normal (0, 1, 0) x (1, 0, 0)
  line L0 (-62, 13.7) -> (-60, 13.7)
  line L1 (-60, 13.7) -> (-60, 19.7)
  line L2 (-60, 19.7) -> (-62, 19.7)
  line L3 (-62, 19.7) -> (-62, 13.7)
  line L4 (-62, 0) -> (-62, 39.4) projected
  line L5 (-62, 0) -> (-46, 0) projected
  line L6 (-75.78, 19.7) -> (20.68, 19.7) projected
  point P0 (0, 0)
  dimension "d86" = 0
  dimension "d87" = 2
  dimension "d96" = 0
  dimension "d97" = 6
  constraints: 8 end point, 2 parallel, 1 horizontal, 1 perpendicular
  measures "d86" distance between parallel lines of L4 L3
  measures "d87" distance between parallel lines of L3 L1
  measures "d96" distance between parallel lines of L2 L6
  measures "d97" distance between parallel lines of L2 L0
extrude "Extrusion14" add sketch "Sketch18" along normal blind 7.6
sketch "Sketch19" plane through (0, 10, 0) normal (0, 1, 0) x (1, 0, 0)
  line L0 (-62, 0) -> (-60, 0)
  line L1 (-60, 0) -> (-60, 19.7)
  line L2 (-60, 19.7) -> (-62, 19.7)
  line L3 (-62, 19.7) -> (-62, 0)
  point P0 (0, 0)
  dimension "d90" = 2
  dimension "d91" = 19.7
  constraints: 8 end point, 2 parallel, 1 horizontal, 1 perpendicular
  measures "d90" distance of L2.end L1.end
  measures "d91" distance between parallel lines of L2 L0
extrude "Extrusion15" add sketch "Sketch19" along normal blind 2
mirror "Mirror5" about plane through (0, 0, -19.7) normal (0, 0, -1) of "Extrusion14", "Extrusion15"
fillet "Fillet8" radius 7 2 edges at (-61, 10, -13.7) (-61, 10, -25.7) curvature continuous yes
fillet "Fillet9" radius 2 2 edges at (-61, 12, 0) (-61, 12, -39.4) curvature continuous yes
equation "\"d24\" = d22 + d42 - d6"
equation "\"d49\" = d48"
equation "\"d60\" = d59"
equation "\"d62\" = d61"
equation "\"d63\" = d61"
equation "\"d64\" = d61"
equation "\"d65\" = d59"
equation "\"d66\" = d59"
equation "\"d72\" = d71"
equation "\"d73\" = 2 * d42"
equation "\"d91\" = d6"
equation "\"d29\" = -d30"
equation "\"d30\" = 19"
body "Solid1"
